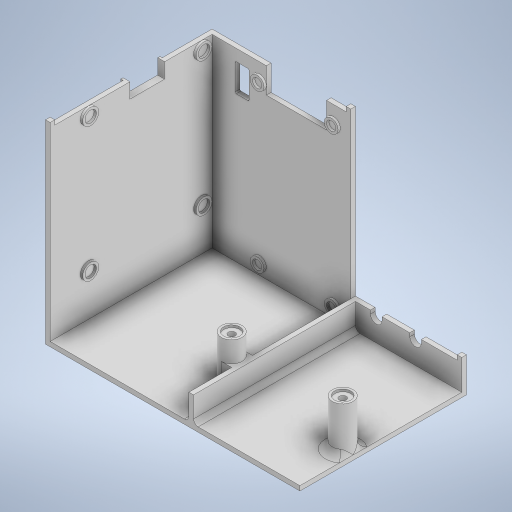
# Autodesk Inventor part: case
Saved by Autodesk Inventor 2024 (Build 280153000, 153)
## iProperties
Created: 2024-04-17
Part Number: case
Material: Generic
Document SubType Name: Modeling
Designer: 22546723
Density: 1 g/cm^3
Appearance: Default
Author: 22546723
## iProperties of the stored document case_3DPrint.ipt
Created: 2024-04-17
Part Number: case_3DPrint
Material: Generic
Document SubType Name: Modeling
Designer: 22546723
Density: 1 g/cm^3
Appearance: Default
Author: 22546723
Autodesk Inventor part; units mm, degrees
ref_plane "YZ Plane" through (0, 0, 0) normal (1, 0, 0) x (0, 1, 0)
ref_plane "XZ Plane" through (0, 0, 0) normal (0, 1, 0) x (-1, 0, 0)
ref_plane "XY Plane" through (0, 0, 0) normal (0, 0, 1) x (1, 0, 0)
sketch "Sketch1" plane through (0, 0, 0) normal (0, 1, 0) x (-1, 0, 0)
  line L0 (58, 35) -> (-50, 35)
  line L1 (-50, 35) -> (-50, -35)
  line L2 (-50, -35) -> (58, -35)
  line L3 (58, -35) -> (58, 35)
  point P0 (0, 0)
  dimension "d1" = 70
  dimension "d129" = 50
  dimension "d130" = 58
  dimension "d131" = 35
  constraints: 8 end point, 2 parallel, 1 horizontal, 1 perpendicular
  measures "d1" distance between parallel lines of L0 L2
  measures "d129" distance from line of L1 point (0, 0)
  measures "d130" distance from line of L3 point (0, 0)
  measures "d131" distance from line of point (0, 0) L2
extrude "Extrusion1" add sketch "Sketch1" along normal blind 2
sketch "Sketch2" plane through (0, 0, 0) normal (0, 1, 0) x (-1, 0, 0)
  line L0 (58, -35) -> (58, 35) projected
  line L1 (58, -35) -> (60, -35)
  line L2 (60, -35) -> (60, 35)
  line L3 (60, 35) -> (58, 35)
  line L4 (58, 35) -> (58, -35)
  point P0 (0, 0)
  dimension "d4" = 2
  constraints: 8 end point, 2 parallel, 1 horizontal, 1 perpendicular, 1 point on line
  measures "d4" distance of L3.end L2.end
extrude "Extrusion2" add sketch "Sketch2" along normal blind 82
sketch "Sketch3" plane through (-58, 2, -35) normal (1, 0, 0) x (0, 0, -1)
  circle A0 centre (-53.5, 18.5) radius 2.5
  circle A1 centre (-4.5, 18.5) radius 2.5
  circle A2 centre (-53.5, 76.5) radius 2.5
  circle A3 centre (-4.5, 76.5) radius 2.5
  line L0 (-70, 0) -> (-70, 80) projected
  line L1 (-70, 0) -> (0, 0) projected
  circle A4 centre (-53.5, 18.5) radius 3.5
  circle A5 centre (-53.5, 76.5) radius 3.5
  circle A6 centre (-4.5, 76.5) radius 3.5
  circle A7 centre (-4.5, 18.5) radius 3.5
  line L2 (-70, 80) -> (0, 80) projected
  line L3 (0, 0) -> (0, 80) projected
  point P0 (-35, -2)
  dimension "d7" = 5
  dimension "d8" = 5
  dimension "d9" = 5
  dimension "d10" = 5
  dimension "d21" = 7
  dimension "d22" = 7
  dimension "d23" = 7
  dimension "d24" = 7
  dimension "d123" = 3.5
  dimension "d124" = 3.5
  dimension "d127" = 4.5
  dimension "d128" = 4.5
  dimension "d155" = 49
  dimension "d156" = 49
  dimension "d157" = 58
  dimension "d159" = 58
  constraints: 8 centre point, 4 coincident
  measures "d7" diameter of A0
  measures "d8" diameter of A1
  measures "d9" diameter of A2
  measures "d10" diameter of A3
  measures "d21" diameter of A4
  measures "d22" diameter of A5
  measures "d23" diameter of A6
  measures "d24" diameter of A7
  measures "d123" distance from line of L2 A2.centre
  measures "d124" distance from line of L2 A3.centre
  measures "d127" distance from line of L3 A3.centre
  measures "d128" distance from line of L3 A1.centre
  measures "d155" distance of A2.centre A3.centre
  measures "d156" distance of A1.centre A0.centre
  measures "d157" distance of A0.centre A2.centre
  measures "d159" distance of A3.centre A1.centre
extrude "Extrusion3" add sketch "Sketch3" along normal blind 1 contours A6 | A5 | A4 | A7
sketch "Sketch4" plane through (0, 2, 0) normal (0, 1, 0) x (1, 0, 0)
  circle A0 centre (45.5, -12) radius 4.5
  circle A1 centre (-2.5, -12) radius 4.5
  line L0 (-58, -35) -> (50, -35) projected
  line L1 (50, -35) -> (50, 35) projected
  point P0 (0, 0)
  dimension "d27" = 9
  dimension "d28" = 9
  dimension "d29" = 23
  dimension "d30" = 23
  dimension "d32" = 48
  constraints: 2 centre point, 1 tangent
  measures "d27" diameter of A0
  measures "d28" diameter of A1
  measures "d29" distance from line of L0 A0.centre
  measures "d30" distance from line of L0 A1.centre
  measures "d32" distance of A0.centre A1.centre
extrude "Extrusion4" add sketch "Sketch4" along normal blind 20
sketch "Sketch5" plane through (-2.5, 22, 12) normal (0, 1, 0) x (1, 0, 0)
  circle A0 centre (0, 0) radius 3.5
  circle A1 centre (0, 0) radius 1.5
  circle A2 centre (0, 0) radius 4.5 projected
  point P0 (2.5, 12)
  dimension "d35" = 7
  dimension "d36" = 3
  constraints: 2 centre point, 1 coincident, 1 concentric
  measures "d35" diameter of A0
  measures "d36" diameter of A1
sketch "Sketch6" plane through (45.5, 22, 12) normal (0, 1, 0) x (1, 0, 0)
  circle A0 centre (0, 0) radius 3.5
  circle A1 centre (0, 0) radius 1.5
  circle A2 centre (0, 0) radius 4.5 projected
  point P0 (-45.5, 12)
  dimension "d37" = 7
  dimension "d38" = 3
  constraints: 2 centre point, 1 coincident, 1 concentric
  measures "d37" diameter of A0
  measures "d38" diameter of A1
extrude "Extrusion5" cut sketch "Sketch5" against normal blind 5 contours A1
extrude "Extrusion6" cut sketch "Sketch6" against normal blind 5 contours A1
extrude "Extrusion9" cut sketch "Sketch5" against normal blind 1 contours A0
extrude "Extrusion10" cut sketch "Sketch6" against normal blind 1 contours A0
sketch "Sketch8" plane through (0, 0, 0) normal (0, 1, 0) x (-1, 0, 0)
  line L0 (-50, -35) -> (60, -35) projected
  line L1 (60, -35) -> (-50, -35)
  line L2 (-50, -35) -> (-50, -37)
  line L3 (-50, -37) -> (60, -37)
  line L4 (60, -37) -> (60, -35)
  point P0 (0, 0)
  dimension "d52" = 2
  constraints: 8 end point, 2 parallel, 1 horizontal, 1 perpendicular, 1 point on line
  measures "d52" distance between parallel lines of L3 L0
extrude "Extrusion11" add sketch "Sketch8" along normal blind 9
sketch "Sketch9" plane through (0, 9, 0) normal (0, 1, 0) x (1, 0, 0)
  line L0 (-58, 35) -> (50, 35) projected
  line L1 (27.5, 37) -> (32.5, 37)
  line L2 (32.5, 37) -> (32.5, 35)
  line L3 (32.5, 35) -> (27.5, 35)
  line L4 (27.5, 35) -> (27.5, 37)
  line L5 (27.5, 37) -> (32.5, 35) construction
  line L6 (32.5, 37) -> (27.5, 35) construction
  line L7 (10.5, 37) -> (15.5, 37)
  line L8 (15.5, 37) -> (15.5, 35)
  line L9 (15.5, 35) -> (10.5, 35)
  line L10 (10.5, 35) -> (10.5, 37)
  line L11 (10.5, 37) -> (15.5, 35) construction
  line L12 (15.5, 37) -> (10.5, 35) construction
  line L13 (50, 37) -> (-60, 37) projected
  circle A0 centre (45.5, -12) radius 4.5 projected
  circle A1 centre (-2.5, -12) radius 4.5 projected
  line L14 (50, 37) -> (2, 37)
  line L15 (2, 37) -> (2, 35)
  line L16 (2, 35) -> (50, 35)
  line L17 (50, 35) -> (50, 37)
  point P0 (0, 0)
  point P1 (30, 36)
  point P2 (13, 36)
  point P3 (13, 37)
  point P4 (30, 37)
  point P5 (2, 36)
  point P6 (2, 37)
  point P7 (10.5, 37)
  point P8 (27.5, 37)
  point P9 (50, 35)
  dimension "d55" = 17
  dimension "d56" = 5
  dimension "d57" = 5
  dimension "d58" = 15.5
  dimension "d59" = 15.5
  dimension "d60" = 4.5
  constraints: 32 end point, 7 midpoint, 6 parallel, 5 point on line, 3 horizontal, 3 perpendicular
  measures "d55" distance of point (30, 36) point (13, 36)
  measures "d56" distance between parallel lines of L8 L10
  measures "d57" distance between parallel lines of L2 L4
  measures "d58" horizontal distance of A0.centre point (30, 36)
  measures "d59" horizontal distance of A1.centre point (13, 36)
  measures "d60" horizontal distance of point (2, 36) A1.centre
extrude "Extrusion12" add sketch "Sketch9" along normal blind 4 contours L15 L13 L10 L0 | L8 L13 L4 L0 | L2 L13 L17 L0
sketch "Sketch10" plane through (0, 9, 0) normal (0, 1, 0) x (1, 0, 0)
  line L0 (-58, 35) -> (-60, 35) projected
  line L1 (2, 37) -> (-60, 37)
  line L2 (-60, 37) -> (-60, 35)
  line L3 (-60, 35) -> (2, 35)
  line L4 (2, 35) -> (2, 37)
  point P0 (0, 0)
  constraints: 8 end point, 2 parallel, 1 horizontal, 1 perpendicular
extrude "Extrusion13" add sketch "Sketch10" along normal blind 73
sketch "Sketch11" plane through (0, 2, 0) normal (0, 1, 0) x (1, 0, 0)
  line L0 (-58, -35) -> (50, -35) projected
  line L1 (2, 35) -> (10.5, 35) projected
  line L2 (2, -35) -> (4, -35)
  line L3 (4, -35) -> (4, 35)
  line L4 (4, 35) -> (2, 35)
  line L5 (2, 35) -> (2, -35)
  circle A0 centre (-2.5, -12) radius 4.5 projected
  point P0 (0, 0)
  dimension "d65" = 2
  constraints: 8 end point, 2 parallel, 2 point on line, 1 horizontal, 1 perpendicular, 1 tangent
  measures "d65" distance of L4.end L3.end
extrude "Extrusion14" add sketch "Sketch11" along normal blind 11 contours L5 L1 L3 L0
sketch "Sketch12" plane through (-58, 2, -35) normal (0, 0, 1) x (1, 0, 0)
  circle A0 centre (52.5, 4.5) radius 2
  circle A1 centre (20.5, 4.5) radius 2
  circle A2 centre (20.5, 72.5) radius 2
  circle A3 centre (52.5, 72.5) radius 2
  line L0 (0, 0) -> (60, 0) projected
  line L1 (60, 11) -> (60, 80) projected
  circle A4 centre (20.5, 72.5) radius 3
  circle A5 centre (52.5, 72.5) radius 3
  circle A6 centre (20.5, 4.5) radius 3
  circle A7 centre (52.5, 4.5) radius 3
  point P0 (58, -2)
  dimension "d68" = 4
  dimension "d69" = 4
  dimension "d70" = 4
  dimension "d71" = 4
  dimension "d72" = 32
  dimension "d73" = 32
  dimension "d74" = 68
  dimension "d75" = 68
  dimension "d76" = 0
  dimension "d77" = 0
  dimension "d78" = 4.5
  dimension "d79" = 7.5
  dimension "d80" = 6
  dimension "d81" = 6
  dimension "d82" = 6
  dimension "d83" = 6
  constraints: 8 centre point, 4 coincident
  measures "d68" diameter of A0
  measures "d69" diameter of A1
  measures "d70" diameter of A2
  measures "d71" diameter of A3
  measures "d72" distance of A0.centre A1.centre
  measures "d73" distance of A3.centre A2.centre
  measures "d74" distance of A1.centre A2.centre
  measures "d75" distance of A0.centre A3.centre
  measures "d76" vertical distance of A0.centre A1.centre
  measures "d77" horizontal distance of A1.centre A2.centre
  measures "d78" distance from line of L0 A1.centre
  measures "d79" distance from line of L1 A3.centre
  measures "d80" diameter of A4
  measures "d81" diameter of A5
  measures "d82" diameter of A6
  measures "d83" diameter of A7
extrude "Extrusion15" add sketch "Sketch12" along normal blind 1
sketch "Sketch13" plane through (0, 82, 0) normal (0, 1, 0) x (1, 0, 0)
  line L0 (10.5, 37) -> (2, 37) projected
  line L1 (2, 35) -> (-58, 35) projected
  line L2 (2, 37) -> (0, 37)
  line L3 (0, 37) -> (0, 35)
  line L4 (0, 35) -> (2, 35)
  line L5 (2, 35) -> (2, 37)
  line L6 (-60, 37) -> (-60, -35) projected
  line L7 (-58, -15) -> (-58, -22) projected
  line L8 (-60, -35) -> (-58, -35)
  line L9 (-58, -35) -> (-58, -33)
  line L10 (-58, -33) -> (-60, -33)
  line L11 (-60, -33) -> (-60, -35)
  point P0 (0, 0)
  point P1 (2, 36)
  point P2 (-50, -33.5)
  dimension "d86" = 2
  dimension "d87" = 2
  constraints: 16 end point, 4 parallel, 2 horizontal, 2 perpendicular, 2 point on line, 1 midpoint
  measures "d86" distance from line of point (2, 36) L3
  measures "d87" distance between parallel lines of L8 L10
extrude "Extrusion16" add sketch "Sketch13" along normal blind 2
sketch "Sketch14" plane through (0, 13, 0) normal (0, 1, 0) x (1, 0, 0)
  line L0 (50, 37) -> (-60, 37) projected
  line L1 (32.5, 35) -> (50, 35) projected
  line L2 (50, 37) -> (48, 37)
  line L3 (48, 37) -> (48, 35)
  line L4 (48, 35) -> (50, 35)
  line L5 (50, 35) -> (50, 37)
  point P0 (0, 0)
  dimension "d90" = 2
  constraints: 8 end point, 2 parallel, 1 horizontal, 1 perpendicular, 1 point on line
  measures "d90" distance of L4.end L3.end
extrude "Extrusion17" add sketch "Sketch14" along normal blind 2
sketch "Sketch15" plane through (50, 0, -37) normal (0, 0, -1) x (-1, 0, 0)
  arc A0 (72.4833, 39.1403) -> (85.5167, 39.1403) centre (79, 34.5) ccw
  line L0 (79, 53.3221) -> (79, 56.8456)
  line L1 (79, 56.952) -> (79, 58.5)
  arc A1 (71.6257, 39.6594) -> (86.3743, 39.6594) centre (79, 34.5) ccw
  arc A2 (79, 58.5) -> (86.3743, 39.6594) centre (121.6175, 64.3173) ccw
  arc A3 (79, 53.3221) -> (85.5167, 39.1403) centre (121.6175, 64.3173) ccw
  arc A4 (71.6257, 39.6594) -> (79, 58.5) centre (36.3825, 64.3173) ccw
  arc A5 (72.4833, 39.1403) -> (79, 53.3221) centre (36.3825, 64.3173) ccw
  arc A6 (78.0006, 31.5344) -> (79.9994, 31.5344) centre (79, 31.5) ccw
  arc A7 (79.9994, 31.5344) -> (79, 44) centre (-57.1211, 26.8139) ccw
  arc A8 (79, 44) -> (78.0006, 31.5344) centre (215.1211, 26.8139) ccw
  line L2 (48, 13) -> (48, 84) projected
  line L3 (0, 0) -> (110, 0) projected
  point P0 (50, 0)
  point P1 (79, 25.5)
  dimension "d93" = 16
  dimension "d94" = 18
  dimension "d97" = 43.0127
  dimension "d98" = 44.013
  dimension "d99" = 2
  dimension "d100" = 0
  dimension "d101" = 3
  dimension "d102" = 12.5
  dimension "d103" = 24
  dimension "d104" = 31
  dimension "d105" = 25.5
  dimension "d106" = 0
  dimension "d107" = 137.2017
  dimension "d108" = 137.2017
  constraints: 21 point on circle, 9 centre point, 4 end point, 4 symmetric about line, 3 coincident, 3 tangent, 2 vertical, 2 other
  measures "d93" diameter of A0
  measures "d94" diameter of A1
  measures "d97" radius of A2
  measures "d98" radius of A3
  measures "d99" diameter of A6
  measures "d100" horizontal distance of A6.centre A0.centre
  measures "d101" distance of A6.centre A0.centre
  measures "d102" distance of A6.centre A7.end
  measures "d103" distance of A0.centre L1.end
  measures "d104" distance from line of L2 A0.centre
  measures "d105" distance from line of point (79, 25.5) L3
  measures "d106" horizontal distance of A6.centre A7.end
  measures "d107" radius of A7
  measures "d108" radius of A8
extrude "Extrusion18" add sketch "Sketch15" along normal blind 1
sketch "Sketch16" plane through (-58, 2, -35) normal (0, 0, 1) x (1, 0, 0)
  line L0 (23.5, 69) -> (49.5, 69)
  line L1 (49.5, 69) -> (49.5, 76)
  line L2 (23.5, 76) -> (23.5, 69)
  line L3 (23.5, 69) -> (49.5, 76) construction
  line L4 (49.5, 69) -> (23.5, 76) construction
  circle A0 centre (20.5, 72.5) radius 2 projected
  circle A1 centre (20.5, 72.5) radius 3 projected
  circle A2 centre (52.5, 72.5) radius 2 projected
  line L5 (23.5, 76) -> (23.5, 80)
  line L6 (0, 80) -> (58, 80) projected
  line L7 (49.5, 76) -> (49.5, 80)
  point P0 (58, -2)
  point P1 (36.5, 72.5)
  point P2 (49.5, 72.5)
  dimension "d112" = 0
  dimension "d113" = 3
  dimension "d114" = 3
  dimension "d115" = 3.5
  constraints: 14 end point, 3 midpoint, 2 parallel, 2 point on line, 1 horizontal, 1 perpendicular, 1 vertical
  measures "d112" vertical distance of A0.centre point (36.5, 72.5)
  measures "d113" distance from line of L2 A1.centre
  measures "d114" distance of A2.centre point (49.5, 72.5)
  measures "d115" distance from line of L0 A0.centre
extrude "Extrusion19" cut sketch "Sketch16" against normal blind 10 contours L2 L5 L6 L7 L1 L0
sketch "Sketch17" plane through (-58, 2, -35) normal (1, 0, 0) x (0, 0, -1)
  line L0 (-35.5, 73.5) -> (-20.5, 73.5)
  line L1 (-20.5, 73.5) -> (-20.5, 80)
  line L2 (-20.5, 80) -> (-35.5, 80)
  line L3 (-35.5, 80) -> (-35.5, 73.5)
  line L4 (-35.5, 73.5) -> (-20.5, 80) construction
  line L5 (-20.5, 73.5) -> (-35.5, 80) construction
  circle A0 centre (-53.5, 76.5) radius 2.5 projected
  circle A1 centre (-4.5, 76.5) radius 2.5 projected
  point P0 (-35, -2)
  point P1 (-28, 76.75)
  dimension "d118" = 15
  dimension "d119" = 25.5
  dimension "d120" = 23.5
  dimension "d121" = 3.5
  dimension "d122" = 3
  constraints: 12 end point, 2 midpoint, 2 parallel, 1 horizontal, 1 perpendicular
  measures "d118" distance of L2.end L1.end
  measures "d119" horizontal distance of point (-28, 76.75) A0.centre
  measures "d120" horizontal distance of A1.centre point (-28, 76.75)
  measures "d121" distance from line of A0.centre L2
  measures "d122" distance from line of A1.centre L0
extrude "Extrusion20" cut sketch "Sketch17" against normal blind 10 contours L3 L2 L1 L0
sketch "Sketch18" plane through (-58, 2, -35) normal (0, 0, 1) x (1, 0, 0)
  line L0 (10, 63) -> (16, 63)
  line L1 (16, 63) -> (16, 75)
  line L2 (16, 75) -> (10, 75)
  line L3 (10, 75) -> (10, 63)
  line L4 (10, 63) -> (16, 75) construction
  line L5 (16, 63) -> (10, 75) construction
  line L6 (0, 80) -> (23.5, 80) projected
  line L7 (0, 0) -> (0, 82) projected
  point P0 (58, -2)
  point P1 (13, 69)
  dimension "d132" = 11
  dimension "d133" = 12
  dimension "d135" = 6
  dimension "d153" = 13
  constraints: 12 end point, 2 midpoint, 2 parallel, 1 horizontal, 1 perpendicular
  measures "d132" distance from line of point (13, 69) L6
  measures "d133" distance between parallel lines of L0 L2
  measures "d135" distance between parallel lines of L1 L3
  measures "d153" distance from line of point (13, 69) L7
extrude "Extrusion21" cut sketch "Sketch18" against normal blind 10
sketch "Sketch19" plane through (-60, 0, -37) normal (-1, 0, 0) x (0, 0, 1)
  line L0 (37.5, 82) -> (70, 82) projected
  line L1 (38.5, 82) -> (38.5, 74.5)
  line L2 (38.5, 74.5) -> (21.5, 74.5)
  line L3 (21.5, 74.5) -> (21.5, 82)
  line L4 (21.5, 80.25) -> (20.5, 80.25)
  line L5 (20.5, 80.25) -> (20.5, 77.25)
  line L6 (20.5, 77.25) -> (21.5, 77.25)
  line L7 (22.5, 75.5) -> (22.5, 82) projected
  line L8 (37.5, 75.5) -> (22.5, 75.5) projected
  line L9 (37.5, 82) -> (37.5, 75.5) projected
  line L10 (0, 82) -> (22.5, 82) projected
  line L11 (21.5, 82) -> (22.5, 82)
  line L12 (22.5, 82) -> (22.5, 75.5)
  line L13 (22.5, 75.5) -> (37.5, 75.5) projected
  line L14 (37.5, 75.5) -> (37.5, 82) projected
  line L15 (37.5, 75.5) -> (37.5, 82)
  line L16 (37.5, 82) -> (38.5, 82)
  line L17 (22.5, 75.5) -> (37.5, 75.5)
  point P0 (37, 0)
  dimension "d138" = 1
  dimension "d139" = 1
  dimension "d140" = 1
  dimension "d141" = 1
  dimension "d142" = 3
  dimension "d143" = 2.75
  constraints: 22 end point, 6 perpendicular, 3 collinear, 3 point on line, 1 horizontal, 1 vertical
  measures "d138" distance between parallel lines of L7 L3
  measures "d139" distance between parallel lines of L2 L8
  measures "d140" distance between parallel lines of L9 L1
  measures "d141" distance between parallel lines of L3 L5
  measures "d142" distance between parallel lines of L6 L4
  measures "d143" distance between parallel lines of L2 L6
extrude "Extrusion22" add sketch "Sketch19" along normal blind 1
fillet "Fillet1" radius 0.5 4 edges at (-48, 65, -36) (-42, 65, -36) (-42, 77, -36) (-48, 77, -36)
fillet "Fillet2" radius 3 1 edges at (41, 2, 12)
fillet "Fillet3" radius 2 1 edges at (4, 2, 0)
sketch "Sketch21" plane through (0, 2, 0) normal (0, 1, 0) x (1, 0, 0)
  circle A0 centre (-2.5, -12) radius 4.5 projected
  line L0 (-2.5, -16.5) -> (2, -16.5)
  line L1 (2, -35) -> (2, -12) projected
  line L2 (-2.5, -7.5) -> (2, -7.5)
  line L3 (2, -7.5) -> (2, -16.5)
  point P0 (0, 0)
  constraints: 6 end point, 2 horizontal, 2 tangent, 1 point on circle, 1 point on line, 1 vertical
extrude "Extrusion23" add sketch "Sketch21" along normal blind 11 contours L1 L0 A0 | A0 L2 L3
fillet "Fillet4" radius 2 4 edges at (-7, 2, 12) (-0.25, 2, 7.5) (-0.25, 2, 16.5) (2, 2, 25.75)
fillet "Fillet5" radius 2.5 4 edges at (15.5, 9, -36) (32.5, 9, -36) (10.5, 9, -36) (27.5, 9, -36)
body "Solid1"
